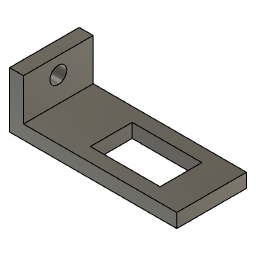
držač kamere (Autodesk Fusion 360 design; units mm, degrees)
Autodesk Fusion 360 part; units mm, degrees
sketch "Sketch1" plane through (0, 0, 0) normal (1, 0, 0) x (0, 1, 0)
  line L0 (12.5, -14) -> (-12.5, -14)
  line L1 (-12.5, -14) -> (-12.5, 6)
  line L2 (-12.5, 6) -> (12.5, 6)
  line L3 (12.5, 6) -> (12.5, -14)
  circle A0 centre (0, 0) radius 3
  dimension "d1" = 25
  dimension "d2" = 20
  dimension "d3" = 6
  dimension "d14" = 6
  constraint horizontal L0
  constraint perpendicular L0 L1
  constraint parallel L0 L2
  constraint parallel L1 L3
  constraint coincident A0.centre origin
  measures "d1" distance of L1.end L2.end
  measures "d2" distance of L0.start L2.end
  measures "d3" diameter of A0
  measures "d14" distance of L2 A0.centre
extrude "Extrude1" add sketch "Sketch1" along normal blind 5
sketch "Sketch2" plane through (5, 0, 0) normal (1, 0, 0) x (0, 1, 0)
  circle A0 centre (0, 0) radius 3
  line L0 (12.5, 6) -> (-12.5, 6)
  line L1 (-12.5, 6) -> (-12.5, -14)
  line L2 (-12.5, -14) -> (12.5, -14)
  line L3 (12.5, -14) -> (12.5, 6)
  line L4 (-12.5, -14) -> (12.5, -14)
  line L5 (12.5, -14) -> (12.5, -9)
  line L6 (12.5, -9) -> (-12.5, -9)
  line L7 (-12.5, -9) -> (-12.5, -14)
  dimension "d6" = 5
  constraint horizontal L4
  constraint vertical L5
  constraint horizontal L6
  constraint vertical L7
  constraint coincident L1.end L2.start
  measures "d6" distance of L1.end L6.end
extrude "Extrude2" add sketch "Sketch2" along normal blind 55 contours L1 L2 L3 L4 L5 L6 L7
sketch "Sketch3" plane through (0, 0, -9) normal (0, 0, 1) x (-1, 0, 0)
  line L0 (-5, -12.5) -> (-5, 12.5)
  line L1 (-5, 12.5) -> (-60, 12.5)
  line L2 (-60, 12.5) -> (-60, -12.5)
  line L3 (-60, -12.5) -> (-5, -12.5)
  line L4 (-49, 7.5) -> (-24, 7.5)
  line L5 (-24, 7.5) -> (-24, -7.5)
  line L6 (-24, -7.5) -> (-49, -7.5)
  line L7 (-49, -7.5) -> (-49, 7.5)
  line L8 (-49, 7.5) -> (-24, -7.5) construction
  line L9 (-24, 7.5) -> (-49, -7.5) construction
  point P0 (-36.5, 0)
  dimension "d9" = 25
  dimension "d10" = 15
  dimension "d13" = 5
  dimension "d15" = 11
  constraint horizontal L4
  constraint perpendicular L4 L5
  constraint parallel L4 L6
  constraint parallel L5 L7
  constraint coincident L8 P0
  constraint coincident L9 P0
  measures "d9" distance of L5.end L6.end
  measures "d10" distance of L4.end L5.end
  measures "d13" distance of L1 L4
  measures "d15" distance of L2 L7
extrude "Extrude3" cut sketch "Sketch3" against normal blind 10 contours L4 L5 L6 L7
